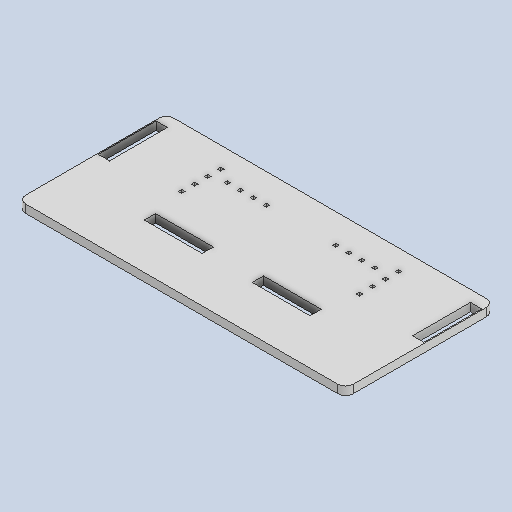
# Autodesk Inventor part: MS_PCB
Saved by Autodesk Inventor 2023 (Build 270158000, 158)
## iProperties
Created: 2024-04-30
Part Number: MS_PCB
Material: Ogólny
Document SubType Name: Modeling
Designer: kamil
Density: 1 g/cm^3
Appearance: Domyślna
Author: kamil
Autodesk Inventor part; units mm, degrees
ref_plane "YZ Plane" through (0, 0, 0) normal (1, 0, 0) x (0, 1, 0)
ref_plane "XZ Plane" through (0, 0, 0) normal (0, 1, 0) x (-1, 0, 0)
ref_plane "XY Plane" through (0, 0, 0) normal (0, 0, 1) x (1, 0, 0)
sketch "Szkic1" plane through (0, 0, 0) normal (0, 1, 0) x (-1, 0, 0)
  line L0 (35.259, 49.5664) -> (-29.741, 49.5664)
  line L1 (-29.741, 49.5664) -> (-29.741, 19.5664)
  line L2 (-29.741, 19.5664) -> (35.259, 19.5664)
  line L3 (35.259, 19.5664) -> (35.259, 49.5664)
  point P0 (0, 0)
  dimension "d0" = 65
  dimension "d1" = 30
  constraints: 8 end point, 2 parallel, 1 horizontal, 1 perpendicular
  measures "d0" distance of L2.end L1.end
  measures "d1" distance of L1.end L0.end
extrude "Wyciągnięcie proste1" add sketch "Szkic1" along normal blind 1.6
fillet "Zaokrąglenie1" radius 2 4 edges at (-35.259, 0.8, 19.5664) (-35.259, 0.8, 49.5664) (29.741, 0.8, 49.5664) (29.741, 0.8, 19.5664)
sketch "Szkic2" plane through (0, 1.6, 0) normal (0, 1, 0) x (1, 0, 0)
  arc A0 (29.741, -21.5664) -> (27.741, -19.5664) centre (27.741, -21.5664) ccw projected
  line L0 (27.741, -19.5664) -> (-33.259, -19.5664) projected
  arc A1 (-33.259, -19.5664) -> (-35.259, -21.5664) centre (-33.259, -21.5664) ccw projected
  line L1 (-35.259, -21.5664) -> (-35.259, -47.5664) projected
  arc A2 (-35.259, -47.5664) -> (-33.259, -49.5664) centre (-33.259, -47.5664) ccw projected
  line L2 (-33.259, -49.5664) -> (27.741, -49.5664) projected
  arc A3 (27.741, -49.5664) -> (29.741, -47.5664) centre (27.741, -47.5664) ccw projected
  line L3 (29.741, -47.5664) -> (29.741, -21.5664) projected
  line L4 (-33.259, -20.0664) -> (27.741, -20.0664)
  arc A4 (29.241, -21.5664) -> (27.741, -20.0664) centre (27.741, -21.5664) ccw
  line L5 (29.241, -21.5664) -> (29.241, -47.5664)
  arc A5 (27.741, -49.0664) -> (29.241, -47.5664) centre (27.741, -47.5664) ccw
  line L6 (27.741, -49.0664) -> (-33.259, -49.0664)
  arc A6 (-34.759, -47.5664) -> (-33.259, -49.0664) centre (-33.259, -47.5664) ccw
  line L7 (-34.759, -47.5664) -> (-34.759, -21.5664)
  arc A7 (-33.259, -20.0664) -> (-34.759, -21.5664) centre (-33.259, -21.5664) ccw
  point P0 (0, 0)
  dimension "d5" = 0.5
  constraints: 8 end point, 8 point on circle, 4 centre point, 7 other
  measures "d5" distance between parallel lines of L0 L4
extrude "Wyciągnięcie proste2" cut sketch "Szkic2" against normal through all
sketch "Szkic3" plane through (0, 1.6, 0) normal (0, 1, 0) x (1, 0, 0)
  line L0 (-19.799, -32.0164) -> (-20.439, -32.0164) projected
  line L1 (-20.439, -32.0164) -> (-20.439, -31.3764) projected
  line L2 (-19.799, -31.3764) -> (-19.799, -32.0164) projected
  line L3 (-20.439, -31.3764) -> (-19.799, -31.3764) projected
  line L4 (-19.799, -29.4764) -> (-20.439, -29.4764) projected
  line L5 (-19.799, -28.8364) -> (-19.799, -29.4764) projected
  line L6 (-20.439, -29.4764) -> (-20.439, -28.8364) projected
  line L7 (-20.439, -28.8364) -> (-19.799, -28.8364) projected
  line L8 (-19.799, -26.9364) -> (-20.439, -26.9364) projected
  line L9 (-19.799, -26.2964) -> (-19.799, -26.9364) projected
  line L10 (-20.439, -26.9364) -> (-20.439, -26.2964) projected
  line L11 (-20.439, -26.2964) -> (-19.799, -26.2964) projected
  line L12 (-20.439, -24.3964) -> (-20.439, -23.7564) projected
  line L13 (-19.799, -24.3964) -> (-20.439, -24.3964) projected
  line L14 (-20.439, -23.7564) -> (-19.799, -23.7564) projected
  line L15 (-19.799, -23.7564) -> (-19.799, -24.3964) projected
  line L16 (-17.469, -25.4431) -> (-16.829, -25.4431) projected
  line L17 (-17.469, -26.0831) -> (-17.469, -25.4431) projected
  line L18 (-16.829, -26.0831) -> (-17.469, -26.0831) projected
  line L19 (-16.829, -25.4431) -> (-16.829, -26.0831) projected
  line L20 (-14.929, -26.0831) -> (-14.929, -25.4431) projected
  line L21 (-14.289, -26.0831) -> (-14.929, -26.0831) projected
  line L22 (-14.929, -25.4431) -> (-14.289, -25.4431) projected
  line L23 (-14.289, -25.4431) -> (-14.289, -26.0831) projected
  line L24 (-12.389, -26.0831) -> (-12.389, -25.4431) projected
  line L25 (-11.749, -26.0831) -> (-12.389, -26.0831) projected
  line L26 (-12.389, -25.4431) -> (-11.749, -25.4431) projected
  line L27 (-11.749, -25.4431) -> (-11.749, -26.0831) projected
  line L28 (-9.849, -26.0831) -> (-9.849, -25.4431) projected
  line L29 (-9.209, -25.4431) -> (-9.209, -26.0831) projected
  line L30 (-9.849, -25.4431) -> (-9.209, -25.4431) projected
  line L31 (-9.209, -26.0831) -> (-9.849, -26.0831) projected
  line L32 (-2.759, -11.5664) -> (-2.759, -67.5664)
  line L33 (-34.259, -33.2664) -> (-32.659, -33.2664) projected
  line L34 (-34.259, -33.2664) -> (-34.259, -22.5664) projected
  line L35 (-34.259, -22.5664) -> (-32.659, -22.5664) projected
  line L36 (-32.659, -22.5664) -> (-32.659, -33.2664) projected
  line L37 (-34.259, -33.2664) -> (-32.659, -33.2664) projected
  line L38 (-7.959, -39.9031) -> (-18.659, -39.9031) projected
  line L39 (-18.659, -39.9031) -> (-18.659, -38.3031) projected
  line L40 (-18.659, -38.3031) -> (-7.959, -38.3031) projected
  line L41 (-7.959, -39.9031) -> (-7.959, -38.3031) projected
  line L42 (2.441, -39.9031) -> (13.141, -39.9031) projected
  line L43 (2.441, -39.9031) -> (2.441, -38.3031) projected
  line L44 (13.141, -38.3031) -> (2.441, -38.3031) projected
  line L45 (13.141, -39.9031) -> (13.141, -38.3031) projected
  line L46 (28.741, -33.2664) -> (28.741, -22.5664) projected
  line L47 (28.741, -33.2664) -> (27.141, -33.2664) projected
  line L48 (27.141, -22.5664) -> (27.141, -33.2664) projected
  line L49 (28.741, -22.5664) -> (27.141, -22.5664) projected
  line L50 (14.281, -32.0164) -> (14.921, -32.0164)
  line L51 (14.921, -32.0164) -> (14.921, -31.3764)
  line L52 (14.281, -31.3764) -> (14.281, -32.0164)
  line L53 (14.921, -31.3764) -> (14.281, -31.3764)
  line L54 (14.281, -29.4764) -> (14.921, -29.4764)
  line L55 (14.281, -28.8364) -> (14.281, -29.4764)
  line L56 (14.921, -29.4764) -> (14.921, -28.8364)
  line L57 (14.921, -28.8364) -> (14.281, -28.8364)
  line L58 (14.281, -26.9364) -> (14.921, -26.9364)
  line L59 (14.281, -26.2964) -> (14.281, -26.9364)
  line L60 (14.921, -26.9364) -> (14.921, -26.2964)
  line L61 (14.921, -26.2964) -> (14.281, -26.2964)
  line L62 (14.921, -24.3964) -> (14.921, -23.7564)
  line L63 (14.281, -24.3964) -> (14.921, -24.3964)
  line L64 (14.921, -23.7564) -> (14.281, -23.7564)
  line L65 (14.281, -23.7564) -> (14.281, -24.3964)
  line L66 (11.951, -25.4431) -> (11.311, -25.4431)
  line L67 (11.951, -26.0831) -> (11.951, -25.4431)
  line L68 (11.311, -26.0831) -> (11.951, -26.0831)
  line L69 (11.311, -25.4431) -> (11.311, -26.0831)
  line L70 (9.411, -26.0831) -> (9.411, -25.4431)
  line L71 (8.771, -26.0831) -> (9.411, -26.0831)
  line L72 (9.411, -25.4431) -> (8.771, -25.4431)
  line L73 (8.771, -25.4431) -> (8.771, -26.0831)
  line L74 (6.871, -26.0831) -> (6.871, -25.4431)
  line L75 (6.231, -26.0831) -> (6.871, -26.0831)
  line L76 (6.871, -25.4431) -> (6.231, -25.4431)
  line L77 (6.231, -25.4431) -> (6.231, -26.0831)
  line L78 (4.331, -26.0831) -> (4.331, -25.4431)
  line L79 (3.691, -25.4431) -> (3.691, -26.0831)
  line L80 (4.331, -25.4431) -> (3.691, -25.4431)
  line L81 (3.691, -26.0831) -> (4.331, -26.0831)
  arc A0 (-33.259, -20.0664) -> (-34.759, -21.5664) centre (-33.259, -21.5664) ccw projected
  line L82 (-34.759, -21.5664) -> (-34.759, -47.5664) projected
  arc A1 (-34.759, -47.5664) -> (-33.259, -49.0664) centre (-33.259, -47.5664) ccw projected
  line L83 (-33.259, -49.0664) -> (27.741, -49.0664) projected
  arc A2 (27.741, -49.0664) -> (29.241, -47.5664) centre (27.741, -47.5664) ccw projected
  line L84 (29.241, -47.5664) -> (29.241, -21.5664) projected
  arc A3 (29.241, -21.5664) -> (27.741, -20.0664) centre (27.741, -21.5664) ccw projected
  line L85 (27.741, -20.0664) -> (-33.259, -20.0664) projected
  line L86 (-32.359, -33.2664) -> (-32.359, -22.2664)
  line L87 (-32.359, -22.2664) -> (-34.559, -22.2664)
  line L88 (-34.559, -22.2664) -> (-34.559, -33.2664)
  line L89 (-34.259, -33.5664) -> (-32.659, -33.5664)
  line L90 (-34.559, -22.2664) -> (-32.359, -22.2664)
  line L91 (-32.359, -22.2664) -> (-32.359, -33.5664)
  line L92 (-32.359, -33.5664) -> (-34.559, -33.5664)
  line L93 (-34.559, -33.5664) -> (-34.559, -22.2664)
  line L94 (-18.959, -40.2031) -> (-7.659, -40.2031)
  line L95 (-7.659, -40.2031) -> (-7.659, -38.0031)
  line L96 (-7.659, -38.0031) -> (-18.959, -38.0031)
  line L97 (-18.959, -38.0031) -> (-18.959, -40.2031)
  line L98 (13.441, -40.2031) -> (2.141, -40.2031)
  line L99 (2.141, -40.2031) -> (2.141, -38.0031)
  line L100 (2.141, -38.0031) -> (13.441, -38.0031)
  line L101 (13.441, -38.0031) -> (13.441, -40.2031)
  line L102 (26.841, -33.5664) -> (29.041, -33.5664)
  line L103 (29.041, -33.5664) -> (29.041, -22.2664)
  line L104 (29.041, -22.2664) -> (26.841, -22.2664)
  line L105 (26.841, -22.2664) -> (26.841, -33.5664)
  point P0 (0, 0)
  dimension "d8" = 0.3
  dimension "d9" = 0.3
  dimension "d10" = 0.3
  dimension "d11" = 0.3
  dimension "d12" = 0.3
  constraints: 106 end point, 32 symmetric about line, 3 parallel, 1 horizontal, 1 perpendicular, 1 point on line, 1 vertical, 13 other
  measures "d8" distance between parallel lines of L36 L86
  measures "d9" distance between parallel lines of L33 L89
  measures "d10" distance between parallel lines of L38 L94
  measures "d11" distance between parallel lines of L42 L98
  measures "d12" distance between parallel lines of L47 L102
extrude "Wyciągnięcie proste3" cut sketch "Szkic3" against normal through all contours L0 L1 L3 L2 | L4 L6 L7 L5 | L8 L10 L11 L9 | L12 L14 L15 L13 | L16 L19 L18 L17 | L20 L22 L23 L21 | L24 L26 L27 L25 | L28 L30 L29 L31 | L34 L35 L36 L33 | L38 L39 L40 L41 | L43 L44 L45 L42 | L47 L48 L49 L46 | L52 L53 L51 L50 | L55 L57 L56 L54 | L59 L61 L60 L58 | L63 L65 L64 L62 | L67 L68 L69 L66 | L71 L73 L72 L70 | L75 L77 L76 L74 | L81 L79 L80 L78 | L91 L92 L89 L93 L88 L87 L86 | L97 L96 L95 L94 | L98 L99 L100 L101 | L105 L104 L103 L102
